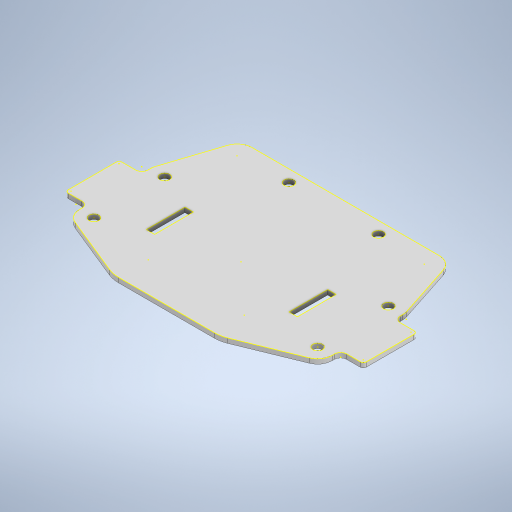
# Autodesk Inventor part: plytka_glowna_v3
Saved by Autodesk Inventor 2023 (Build 270158000, 158)
## iProperties
Created: 2024-04-28
Part Number: plytka_glowna_v3
Material: Ogólny
Document SubType Name: Modeling
Designer: kamil
Density: 1 g/cm^3
Appearance: Domyślna
Author: kamil
Autodesk Inventor part; units mm, degrees
ref_plane "YZ Plane" through (0, 0, 0) normal (1, 0, 0) x (0, 1, 0)
ref_plane "XZ Plane" through (0, 0, 0) normal (0, 1, 0) x (-1, 0, 0)
ref_plane "XY Plane" through (0, 0, 0) normal (0, 0, 1) x (1, 0, 0)
sketch "Szkic1" plane through (0, 0, 0) normal (0, 1, 0) x (-1, 0, 0)
  arc A0 (49.9, 8) -> (48.9, 9) centre (48.9, 8) ccw
  line L0 (48.9, 9) -> (44.3, 9)
  arc A1 (42.3, 11) -> (44.3, 9) centre (44.3, 11) ccw
  line L1 (42.3, 11) -> (42.3, 11.85)
  arc A2 (42.3, 11.85) -> (39.1714, 16.3842) centre (37.45, 11.85) ccw
  line L2 (39.1714, 16.3842) -> (18, 25)
  line L3 (18, 25) -> (-18, 25)
  line L4 (-18, 25) -> (-39.1714, 16.3842)
  arc A3 (-39.1714, 16.3842) -> (-42.3, 11.85) centre (-37.45, 11.85) ccw
  line L5 (-42.3, 11.85) -> (-42.3, 11)
  arc A4 (-44.3, 9) -> (-42.3, 11) centre (-44.3, 11) ccw
  line L6 (-44.3, 9) -> (-48.9, 9)
  arc A5 (-48.9, 9) -> (-49.9, 8) centre (-48.9, 8) ccw
  line L7 (-49.9, 8) -> (-49.9, -8)
  arc A6 (-49.9, -8) -> (-48.9, -9) centre (-48.9, -8) ccw
  line L8 (-48.9, -9) -> (-44.3, -9)
  arc A7 (-42.3, -11) -> (-44.3, -9) centre (-44.3, -11) ccw
  line L9 (-42.3, -11) -> (-42.3, -11.85)
  arc A8 (-42.3, -11.85) -> (-42.0609, -13.3541) centre (-37.45, -11.85) ccw
  line L10 (-42.0609, -13.3541) -> (-36.1252, -31.5506)
  arc A9 (-36.1252, -31.5506) -> (-31.3717, -35) centre (-31.3717, -30) ccw
  line L11 (-31.3717, -35) -> (31.3717, -35)
  arc A10 (31.3717, -35) -> (36.1252, -31.5506) centre (31.3717, -30) ccw
  line L12 (36.1252, -31.5506) -> (42.0609, -13.3541)
  arc A11 (42.0609, -13.3541) -> (42.3, -11.85) centre (37.45, -11.85) ccw
  line L13 (42.3, -11.85) -> (42.3, -11)
  arc A12 (44.3, -9) -> (42.3, -11) centre (44.3, -11) ccw
  line L14 (44.3, -9) -> (48.9, -9)
  arc A13 (48.9, -9) -> (49.9, -8) centre (48.9, -8) ccw
  line L15 (49.9, -8) -> (49.9, 8)
  line L16 (25.3, -6.4859) -> (22.5, -6.4859)
  line L17 (22.5, -6.4859) -> (22.5, 6.4859)
  line L18 (22.5, 6.4859) -> (25.3, 6.4859)
  line L19 (25.3, 6.4859) -> (25.3, -6.4859)
  circle A14 centre (37.45, 11.85) radius 1.6
  circle A15 centre (37.45, -11.85) radius 1.6
  circle A16 centre (15, -31) radius 1.6
  circle A17 centre (-15, -31) radius 1.6
  circle A18 centre (-37.45, 11.85) radius 1.6
  circle A19 centre (-37.45, -11.85) radius 1.6
  line L20 (-25.3, -6.4859) -> (-25.3, 6.4859)
  line L21 (-25.3, 6.4859) -> (-22.5, 6.4859)
  line L22 (-22.5, 6.4859) -> (-22.5, -6.4859)
  line L23 (-22.5, -6.4859) -> (-25.3, -6.4859)
  point P0 (0, 0)
  point P1 (0, 0)
  point P2 (0, -35)
  point P3 (0, 25)
  dimension "d0" = 36
  dimension "d1" = 60
  constraints: 48 end point, 28 point on circle, 20 centre point, 9 horizontal, 9 vertical, 2 midpoint, 1 vertical alignment, 68 other
  measures "d0" distance of L2.end L3.end
  measures "d1" distance between parallel lines of L3 L11
extrude "Wyciągnięcie proste1" add sketch "Szkic1" along normal blind 1.6
fillet "Zaokrąglenie1" radius 10 2 edges at (-18, 0.8, 25) (18, 0.8, 25)
sketch "Szkic2" plane through (0, 1.6, 0) normal (0, 1, 0) x (1, 0, 0)
  arc A0 (16.0432, -25) -> (19.8125, -24.2624) centre (16.0432, -15) ccw projected
  line L0 (19.8125, -24.2624) -> (39.1714, -16.3842) projected
  arc A1 (39.1714, -16.3842) -> (42.3, -11.85) centre (37.45, -11.85) ccw projected
  line L1 (42.3, -11.85) -> (42.3, -11) projected
  arc A2 (44.3, -9) -> (42.3, -11) centre (44.3, -11) ccw projected
  line L2 (44.3, -9) -> (48.9, -9) projected
  arc A3 (48.9, -9) -> (49.9, -8) centre (48.9, -8) ccw projected
  line L3 (49.9, -8) -> (49.9, 8) projected
  arc A4 (49.9, 8) -> (48.9, 9) centre (48.9, 8) ccw projected
  line L4 (48.9, 9) -> (44.3, 9) projected
  arc A5 (42.3, 11) -> (44.3, 9) centre (44.3, 11) ccw projected
  line L5 (42.3, 11) -> (42.3, 11.85) projected
  arc A6 (42.3, 11.85) -> (42.0609, 13.3541) centre (37.45, 11.85) ccw projected
  line L6 (42.0609, 13.3541) -> (36.1252, 31.5506) projected
  arc A7 (36.1252, 31.5506) -> (31.3717, 35) centre (31.3717, 30) ccw projected
  line L7 (31.3717, 35) -> (-31.3717, 35) projected
  arc A8 (-31.3717, 35) -> (-36.1252, 31.5506) centre (-31.3717, 30) ccw projected
  line L8 (-36.1252, 31.5506) -> (-42.0609, 13.3541) projected
  arc A9 (-42.0609, 13.3541) -> (-42.3, 11.85) centre (-37.45, 11.85) ccw projected
  line L9 (-42.3, 11.85) -> (-42.3, 11) projected
  arc A10 (-44.3, 9) -> (-42.3, 11) centre (-44.3, 11) ccw projected
  line L10 (-44.3, 9) -> (-48.9, 9) projected
  arc A11 (-48.9, 9) -> (-49.9, 8) centre (-48.9, 8) ccw projected
  line L11 (-49.9, 8) -> (-49.9, -8) projected
  arc A12 (-49.9, -8) -> (-48.9, -9) centre (-48.9, -8) ccw projected
  line L12 (-48.9, -9) -> (-44.3, -9) projected
  arc A13 (-42.3, -11) -> (-44.3, -9) centre (-44.3, -11) ccw projected
  line L13 (-42.3, -11) -> (-42.3, -11.85) projected
  arc A14 (-42.3, -11.85) -> (-39.1714, -16.3842) centre (-37.45, -11.85) ccw projected
  line L14 (-39.1714, -16.3842) -> (-19.8125, -24.2624) projected
  arc A15 (-19.8125, -24.2624) -> (-16.0432, -25) centre (-16.0432, -15) ccw projected
  line L15 (-16.0432, -25) -> (16.0432, -25) projected
  circle A16 centre (-37.45, -11.85) radius 1.6 projected
  circle A17 centre (37.45, -11.85) radius 1.6 projected
  circle A18 centre (15, 31) radius 1.6 projected
  circle A19 centre (-15, 31) radius 1.6 projected
  circle A20 centre (-37.45, 11.85) radius 1.6 projected
  circle A21 centre (37.45, 11.85) radius 1.6 projected
  line L16 (22.5, -6.4859) -> (22.5, 6.4859) projected
  line L17 (22.5, 6.4859) -> (25.3, 6.4859) projected
  line L18 (25.3, 6.4859) -> (25.3, -6.4859) projected
  line L19 (25.3, -6.4859) -> (22.5, -6.4859) projected
  line L20 (-22.5, -6.4859) -> (-25.3, -6.4859) projected
  line L21 (-25.3, -6.4859) -> (-25.3, 6.4859) projected
  line L22 (-25.3, 6.4859) -> (-22.5, 6.4859) projected
  line L23 (-22.5, 6.4859) -> (-22.5, -6.4859) projected
  point P0 (0, 0)
